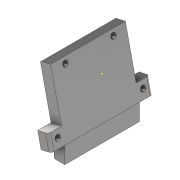
# Autodesk Inventor part: Cover of robot upper base
Saved by Autodesk Inventor 2020.3 (Build 243373010, 373A)
## iProperties
Created: 2021-04-28
Part Number: Cover of robot upper base
Material: Steel, Alloy
Document SubType Name: Modeling
Designer: marti
Density: 7.73 g/cm^3
Appearance: Semi-Polished
Author: marti
Autodesk Inventor part; units mm, degrees
ref_plane "YZ Plane" through (0, 0, 0) normal (1, 0, 0) x (0, 1, 0)
ref_plane "XZ Plane" through (0, 0, 0) normal (0, 1, 0) x (-1, 0, 0)
ref_plane "XY Plane" through (0, 0, 0) normal (0, 0, 1) x (1, 0, 0)
sketch "Sketch9" plane through (0, 0, 0) normal (0, 0, 1) x (1, 0, 0)
  line L0 (38.6921, -112.9498) -> (20.6921, -112.9498)
  arc A0 (18.6921, -110.9498) -> (20.6921, -112.9498) centre (20.6921, -110.9498) ccw
  line L1 (18.6921, -110.9498) -> (18.6921, -83.6655)
  line L2 (-0.9314, 4.1691) -> (18.6921, -83.6655)
  line L3 (-6.8342, 30.5897) -> (0, 0)
  arc A1 (-5.3184, 32.9777) -> (-6.8342, 30.5897) centre (-4.8823, 31.0258) ccw
  line L4 (12.2485, 36.9024) -> (-5.3184, 32.9777)
  line L5 (38.6921, -112.9498) -> (38.6921, -81.4586)
  line L6 (38.6921, -81.4586) -> (12.2485, 36.9024)
  point P0 (0, 0)
  constraints: 14 end point, 4 point on circle, 2 centre point
extrude "Extrusion8" add sketch "Sketch9" along normal mid plane 190
sketch "Sketch10" plane through (38.6921, -112.9498, 95) normal (1, 0, 0) x (0, 0, -1)
  point P0 (95, 112.9498)
sketch "Sketch11" plane through (0, 0, 0) normal (1, 0, 0) x (0, 1, 0)
  line L0 (-112.9498, 70) -> (-81.4586, 70)
  line L1 (-112.9498, -70) -> (-81.4586, -70)
  line L2 (-81.4586, -95) -> (-81.4586, 95) projected
  line L3 (-112.9498, 95) -> (-81.4586, 95) projected
  line L4 (-112.9498, -95) -> (-112.9498, 95) projected
  line L5 (-81.4586, -95) -> (-112.9498, -95) projected
  point P0 (0, 0)
  dimension "d39" = 140
  dimension "d40" = 70
  constraints: 4 end point, 4 point on line, 2 horizontal
  measures "d39" distance between parallel lines of L0 L1
  measures "d40" distance from line of point (0, 0) L0
extrude "Extrusion9" cut sketch "Sketch11" along normal through all both and the other way through all contours L4 L3 L2 L0 | L1 L2 L5 L4
sketch "Sketch12" plane through (12.2485, 36.9024, 95) normal (0.97594, 0.2180394, 0) x (0, 0, -1)
  line L0 (25, -121.279) -> (25, 0)
  line L1 (165, -121.279) -> (165, 0)
  line L2 (190, 0) -> (190, -121.279) projected
  line L3 (0, -121.279) -> (0, 0) projected
  line L4 (190, 0) -> (0, 0) projected
  line L5 (0, -121.279) -> (0, 0) projected
  line L6 (25, -121.279) -> (0, -121.279) projected
  line L7 (165, -121.279) -> (25, -121.279) projected
  line L8 (190, -121.279) -> (165, -121.279) projected
  line L9 (190, 0) -> (190, -121.279) projected
  point P0 (95, -33.3439)
  dimension "d44" = 25
  dimension "d45" = 25
  dimension "d46" = 140
  constraints: 4 end point, 4 point on line, 2 vertical
  measures "d44" distance between parallel lines of L1 L2
  measures "d45" distance between parallel lines of L0 L3
  measures "d46" distance between parallel lines of L1 L0
extrude "Extrusion10" cut sketch "Sketch12" along normal through all both and the other way through all contours L6 L3 L4 L0 | L1 L4 L2 L8
sketch "Sketch13" plane through (12.2485, 36.9024, 70) normal (0.97594, 0.2180394, 0) x (0, 0, -1)
  line L0 (140, -152.0125) -> (0, -152.0125) projected
  line L1 (70, -152.0125) -> (70, -0.0751)
  circle A0 centre (115, -10.33) radius 3.4585
  circle A1 centre (25, -10.33) radius 3.4585
  circle A2 centre (-10, -105.33) radius 3.4585
  circle A3 centre (150, -105.33) radius 3.4585
  line L2 (0, 0) -> (140, 0)
  line L3 (0, 0) -> (0, -31.3439)
  line L4 (0, -31.3439) -> (12.5, -31.3439)
  line L5 (12.5, -31.3439) -> (12.5, -72.33)
  line L6 (12.5, -72.33) -> (0, -72.33)
  line L7 (0, -72.33) -> (0, -92.33)
  line L8 (-25, -92.33) -> (0, -92.33)
  ellipse E0 centre (2, -126.2447) end of major axis (2, -117.072) minor radius 2 (2, -117.072) -> (0.6988, -119.279) ccw
  line L9 (2, -117.072) -> (27.5, -117.072)
  line L10 (27.5, -27.072) -> (27.5, -117.072)
  line L11 (112.5, -27.072) -> (27.5, -27.072)
  line L12 (112.5, -117.072) -> (112.5, -27.072)
  line L13 (112.5, -117.072) -> (138, -117.072)
  ellipse E1 centre (138, -126.2447) end of major axis (138, -135.4173) minor radius 2 (139.3012, -119.279) -> (138, -117.072) ccw
  line L14 (165, -92.33) -> (165, -114.8107)
  line L15 (140, -92.33) -> (165, -92.33)
  line L16 (140, -92.33) -> (140, -72.33)
  line L17 (140, -72.33) -> (127.5, -72.33)
  line L18 (127.5, -72.33) -> (127.5, -31.3439)
  line L19 (127.5, -31.3439) -> (140, -31.3439)
  line L20 (140, -31.3439) -> (140, 0)
  line L21 (0, 0) -> (0, -121.279) projected
  line L22 (140, -121.279) -> (140, 0) projected
  line L23 (0, -121.279) -> (0, -152.0125) projected
  line L24 (0, -121.279) -> (-25, -121.279)
  line L25 (-25, -92.33) -> (-25, -121.279)
  line L26 (-25, -92.33) -> (7.4202, -92.33) construction
  line L27 (140, -121.279) -> (165, -121.279)
  line L28 (165, -92.33) -> (165, -121.279)
  point P0 (70, -33.3439)
  point P1 (-25.1048, -117.072)
  point P2 (-25, -119.279)
  point P3 (165, -119.279)
  dimension "d58" = 90
  constraints: 50 end point, 4 centre point, 3 point on line, 2 horizontal, 2 vertical, 1 midpoint, 8 other
  measures "d58" angle of L25 L26
extrude "Extrusion11" add sketch "Sketch13" against normal up to surface (20 mm away) contours A2 | A3 | L8 L21 L24 L25 | L14 L28 L27 L22 L15
hole "Hole1" at (35.2146, -65.8933, -80) at (14.5009, 26.8209, -45) at (14.5009, 26.8209, 45) at (35.2146, -65.8933, 80) direction (-0.97594, -0.2180394, 0) diameter 6.917 depth 27.125 tip angle 118 counterbore diameter 10.025 counterbore depth 6.025 thread size "M8x1" class "6H" standard "ISO Metric profile"
fillet "Fillet3" radius 5 2 edges at (35.5361, -67.3324, 95) (35.5361, -67.3324, -95)
equation "\"d40\" = 0.5 * d39"
body "Solid4"
